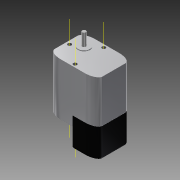
# Autodesk Inventor part: 12V geared motor
Saved by Autodesk Inventor 2013 (Build 170138000, 138)
## iProperties
Created: 2015-01-05
Part Number: 12V geared motor
Material: Generic
Document SubType Name: Modeling
Designer: Nico
Density: 1 g/cm^3
Author: Nico
Autodesk Inventor part; units mm, degrees
ref_plane "YZ Plane" through (0, 0, 0) normal (1, 0, 0) x (0, 1, 0)
ref_plane "XZ Plane" through (0, 0, 0) normal (0, 1, 0) x (-1, 0, 0)
ref_plane "XY Plane" through (0, 0, 0) normal (0, 0, 1) x (1, 0, 0)
sketch "Sketch1" plane through (0, 0, 0) normal (0, 0, 1) x (1, 0, 0)
  ellipse E0 centre (10, 24) end of major axis (0, 24) minor radius 5 (10, 29) -> (0, 24) ccw
  ellipse E1 centre (30, 24) end of major axis (40, 24) minor radius 5 (40, 24) -> (30, 29) ccw
  ellipse E2 centre (30, 5) end of major axis (40, 5) minor radius 5 (30, 0) -> (40, 5) ccw
  ellipse E3 centre (10, 5) end of major axis (0, 5) minor radius 5 (0, 5) -> (10, 0) ccw
  line L0 (30, 29) -> (10, 29)
  line L1 (0, 24) -> (0, 5)
  line L2 (10, 0) -> (30, 0)
  line L3 (40, 5) -> (40, 24)
  point P0 (0, 0)
  constraints: 8 end point, 2 parallel, 1 horizontal, 1 perpendicular, 16 other
extrude "Extrusion2" add sketch "Sketch1" along normal blind 36
sketch "Sketch2" plane through (0, 0, 36) normal (0, 0, 1) x (1, 0, 0)
  line L0 (0, 24) -> (0, 5) projected
  line L1 (10, 0) -> (30, 0) projected
  line L2 (30, 29) -> (10, 29) projected
  line L3 (14.358, 14.5) -> (-3.5199, 14.5)
  circle A0 centre (3, 14.5) radius 1.5
  line L4 (21.3512, 2.5) -> (5.4191, 2.5)
  line L5 (21.3512, 26.5) -> (5.4191, 26.5)
  line L6 (19.5, 31.1643) -> (19.5, -4.236)
  circle A1 centre (19.5, 26.5) radius 1.5001
  circle A2 centre (19.5, 2.5) radius 1.5001
  point P0 (0, 0)
  dimension "d16" = 29
  dimension "d17" = 14.5
  dimension "d18" = 3
  dimension "d19" = 3
  dimension "d20" = 24
  dimension "d21" = 12
  dimension "d22" = 16.5
  constraints: 8 end point, 5 point on line, 3 centre point, 3 parallel, 1 perpendicular
  measures "d16" distance between parallel lines of L2 L1
  measures "d17" distance between parallel lines of L1 L3
  measures "d18" diameter of A0
  measures "d19" distance from line of L0 A0.centre
  measures "d20" distance between parallel lines of L5 L4
  measures "d21" distance between parallel lines of L4 L3
  measures "d22" distance from line of L6 A0.centre
extrude "Extrusion3" cut sketch "Sketch2" against normal blind 5
thread "Thread1" size "M3x0.5" class "6H" standard "ANSI Metric M Profile" full length
thread "Thread2" size "M3x0.5" class "6H" standard "ANSI Metric M Profile" full length
thread "Thread3" size "M3x0.5" class "6H" standard "ANSI Metric M Profile" full length
sketch "Sketch3" plane through (0, 0, 36) normal (0, 0, 1) x (1, 0, 0)
  line L0 (0, 24) -> (0, 5) projected
  line L1 (30, 29) -> (10, 29) projected
  line L2 (-1.3483, 17.5) -> (17.9999, 17.5)
  line L3 (12, 35.2177) -> (12, 13)
  circle A0 centre (10.5, 19) radius 1.5
  point P0 (0, 0)
  dimension "d31" = 11.5
  dimension "d32" = 12
  dimension "d33" = 3
  dimension "d34" = 1.5
  dimension "d35" = 1.5
  constraints: 4 end point, 1 centre point, 1 parallel, 1 perpendicular
  measures "d31" distance between parallel lines of L2 L1
  measures "d32" distance between parallel lines of L3 L0
  measures "d33" diameter of A0
  measures "d34" distance from line of L2 A0.centre
  measures "d35" distance from line of L3 A0.centre
extrude "Extrusion4" add sketch "Sketch3" along normal blind 11 contours A0
sketch "Sketch4" plane through (0, 0, 36) normal (0, 0, 1) x (1, 0, 0)
  circle A0 centre (10.5, 19) radius 1.5 projected
  circle A1 centre (10.5, 19) radius 5
  point P0 (0, 0)
  dimension "d40" = 10
  constraints: 1 centre point, 1 coincident
  measures "d40" diameter of A1
extrude "Extrusion5" add sketch "Sketch4" along normal blind 0.67
sketch "Sketch5" plane through (0, 0, 0) normal (0, 0, -1) x (-1, 0, 0)
  ellipse E0 centre (-10, 24) end of major axis (0, 24) minor radius 5 (0, 24) -> (-10, 29) ccw projected
  line L0 (-30, 29) -> (-10, 29) projected
  line L1 (-40, 5) -> (-40, 24) projected
  line L2 (-10, 0) -> (-30, 0) projected
  ellipse E1 centre (-10, 5) end of major axis (0, 5) minor radius 5 (-10, 0) -> (0, 5) ccw projected
  line L3 (0, 24) -> (0, 5) projected
  line L4 (-20, 29) -> (-20, 0)
  point P0 (0, 0)
  dimension "d42" = 40
  dimension "d43" = 20
  constraints: 2 end point, 2 midpoint, 2 other
  measures "d42" distance between parallel lines of L1 L3
  measures "d43" distance between parallel lines of L4 L3
extrude "Extrusion6" add sketch "Sketch5" along normal blind 8
sketch "Sketch6" plane through (0, 0, 0) normal (0, 0, -1) x (-1, 0, 0)
  line L0 (-20, 0) -> (-20, 29) projected
  line L1 (-30, 29) -> (-20, 29) projected
  ellipse E0 centre (-30, 24) end of major axis (-40, 24) minor radius 5 (-30, 29) -> (-40, 24) ccw projected
  line L2 (-40, 5) -> (-40, 24) projected
  ellipse E1 centre (-30, 5) end of major axis (-40, 5) minor radius 5 (-40, 5) -> (-30, 0) ccw projected
  line L3 (-20, 0) -> (-30, 0) projected
  point P0 (0, 0)
  constraints: 2 other
fillet "Fillet2" radius 0.5 13 edges at (15, 29, -8) (0, 14.5, -8) (2.9289, 1.4645, -8) (15, 0, -8) (2.9289, 27.5355, -8) (20, 29, -4) (37.0711, 27.5355, 0) (40, 14.5, 0) (37.0711, 1.4645, 0) (25, 0, 0) (25, 29, 0) (20, 14.5, -8) (20, 0, -4)
extrude "Extrusion8" add sketch "Sketch6" along normal blind 24
fillet "Fillet3" radius 2 6 edges at (25, 0, -24) (40, 14.5, -24) (37.0711, 27.5355, -24) (25, 29, -24) (37.0711, 1.4645, -24) (20, 14.5, -24)
body "Solid2"
